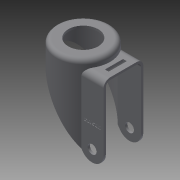
# Autodesk Inventor part: 2.05456.444-FORK
Saved by Autodesk Inventor 2014 SP2 (Build 180246200, 246)
## iProperties
Created: 2018-12-09
Part Number: 2.05456.444-FORK
Material: Generic
Catalog Web Link: www.cadenas.de
Description: 2 Series Stainless Steel Fork-Capacitiy up to 325 lbs Each
Vendor: COLSONGROUP
Document SubType Name: Modeling
Designer: psadmin
Manufacturer: COLSONGROUP
Mass: 30.1099 g
Surface Area: 255.342 cm^2
Volume: 30.1099 cm^3
Density: 1 g/cm^3
Appearance: PSOLRGB-175-175-175
Category: PARTsolutions
Company: COLSONGROUP
Title: 2.05456.444-FORK
Author: Cadenas PARTsolutions
Comments: Capacitiy up to 325 lbs Each
PSOL_IDENT_0: {$CADENAS_DATA\23d-libs\colsongroup\colson\casters\2_series_stainless_steel\2_series_stainless_steel
PSOL_IDENT_1: _fork.prj},210 {VTYP=3D},{NB=2.05456.444-FORK},{LINA=2.05456.444-FORK},{NN=2 Series Stainless Steel
PSOL_IDENT_2: Fork},{DATE=13.07.2017 07:15:58},{GEOMDATE=28.02.2017 12:04:00},{VERSION=},{LINEID=10},{WBVAR=MO,D,W
PSOL_IDENT_3: ,TT,BR},{WBNUMERIC=D,W}  {NB=2.05456.444-FORK},{LINA=2.05456.444-FORK},{KT=DUMMY},{PN=2.05456.444},{
PSOL_IDENT_4: SER=2 Series Stainless Steel},{MO=TPS},{MOPN=456},{SIZE=3 3/4\" x 2 3/4\"},{D=5.00000000},{DALG=3,3.
PSOL_IDENT_5: 5,4,5},{DPN=05},{W=1.25},{WALG=1.25,1.3125},{TT=PRFG},{TTALG= 'THT','ThermoTech', 'PLF','Polyolefin'
PSOL_IDENT_6: ,'PHI','Polyurethane HI-TECH','TPE','TPE High-Temp','PRFG','Performa Rubber (Flat)','TH','Thermo' },
PSOL_IDENT_7: {WTPN1=4},{WTPN3=},{WB=Derlin},{WBPN=44},{CAP=325},{BR=},{BRALG= '','None',' BRK1','Top Lock Brake (
PSOL_IDENT_8: BRK1)',' BRK2','Tech Lock Brake (BRK2)',' BRK4','Total Lock Brake (BRK4)' },{H=6.18750000},{R=4.0625
PSOL_IDENT_9: 0000},{WEIGHT=2.75000000},{FONTSIZE=0.12375},{MODEL=Swivel},{HEIGHT=2.75000},{WIDTH=3.75000},{HDY1=2
PSOL_IDENT_10: .81250},{HDY2=3.06250},{HDX1=1.75000},{HR=0.17000},{RR=0.5},{CP=0.53600},{X=1.25},{Y=-2.1515}
NN: 2 Series Stainless Steel Fork
NT: Capacitiy up to 325 lbs Each
NB: 2.05456.444-FORK
NBSYN: $PN.-FORK
LINA: 2.05456.444-FORK
SER: 2 Series Stainless Steel
MO: Top Plate Swivel
D: 5
W: 1.25
TT: Performa Rubber (Flat)
HDY1: 2.8125
HDY2: 3.0625
HDX1: 1.75
HR: 0.17
SUPPLIER: COLSONGROUP
ARTICLENO: 2.05456.444-FORK
BOMINFO: 2.05456.444-FORK
CREATOR: CADENAS GmbH
Autodesk Inventor part; units mm, degrees
sketch "Sketch_9" plane through (0, 0, 0) normal (1, 0, 0) x (0, 1, 0)
  line L0 (-15.494, 21.971) -> (-139.3508, 21.971)
  line L1 (-139.3508, 21.971) -> (-139.3508, -21.971)
  line L2 (-139.3508, -21.971) -> (-15.494, -21.971)
  arc A0 (-15.494, -21.971) -> (-8.382, -14.859) centre (-15.494, -14.859) ccw
  line L3 (-8.382, -14.859) -> (-8.382, 14.859)
  arc A1 (-8.382, 14.859) -> (-15.494, 21.971) centre (-15.494, 14.859) ccw
  constraints: 8 end point, 4 point on circle, 2 centre point
extrude "Extrusion1" add sketch "Sketch_9" along normal blind 45.72
sketch "Sketch_10" plane through (0, 0, 0) normal (0, 0, 1) x (1, 0, 0)
  line L0 (0, 0) -> (0, -130.9688)
  line L1 (0, -130.9688) -> (-29.591, -130.9688)
  line L2 (-29.591, -130.9688) -> (-29.591, -4.826)
  arc A0 (-24.765, 0) -> (-29.591, -4.826) centre (-24.765, -4.826) ccw
  line L3 (-24.765, 0) -> (0, 0)
  line L4 (0, 0) -> (0, -130.9688)
  constraints: 10 end point, 2 point on circle, 1 centre point
revolve "Revolution1" add sketch "Sketch_10" angle 360 about axis through (0, 0, 0) along (0, 1, 0)
sketch "Sketch_11" plane through (0, 0, 0) normal (0, 0, 1) x (1, 0, 0)
  line L0 (0, 0) -> (0, -130.9688)
  line L1 (0, -130.9688) -> (-27.051, -130.9688)
  line L2 (-27.051, -130.9688) -> (-27.051, -4.826)
  arc A0 (-24.765, -2.54) -> (-27.051, -4.826) centre (-24.765, -4.826) ccw
  line L3 (-24.765, -2.54) -> (-16.51, -2.54)
  line L4 (-16.51, -2.54) -> (-16.51, 0)
  line L5 (-16.51, 0) -> (0, 0)
  line L6 (0, 0) -> (0, -130.9688)
  constraints: 14 end point, 2 point on circle, 1 centre point
revolve "Revolution2" cut sketch "Sketch_11" angle 360 about axis through (0, 0, 0) along (0, 1, 0)
sketch "Sketch_12" plane through (0, 0, 0) normal (1, 0, 0) x (0, 1, 0)
  line L0 (-15.494, 19.431) -> (-141.8907, 19.431)
  line L1 (-141.8907, 19.431) -> (-141.8907, -19.431)
  line L2 (-141.8907, -19.431) -> (-15.494, -19.431)
  arc A0 (-15.494, -19.431) -> (-10.922, -14.859) centre (-15.494, -14.859) ccw
  line L3 (-10.922, -14.859) -> (-10.922, 14.859)
  arc A1 (-10.922, 14.859) -> (-15.494, 19.431) centre (-15.494, 14.859) ccw
  constraints: 8 end point, 4 point on circle, 2 centre point
extrude "Extrusion2" cut sketch "Sketch_12" along normal blind 50.8
sketch "Sketch_13" plane through (0, 0, 0) normal (0, 0, 1) x (1, 0, 0)
  line L0 (-42.291, -171.3865) -> (84.709, -171.3865)
  line L1 (84.709, -171.3865) -> (84.709, 0)
  line L2 (84.709, 0) -> (44.45, 0)
  line L3 (44.45, 0) -> (44.45, -80.0481)
  arc A0 (21.3298, -87.3083) -> (44.45, -80.0481) centre (31.75, -80.0481) ccw
  line L4 (21.3298, -87.3083) -> (-29.591, -14.224)
  line L5 (-29.591, -14.224) -> (-42.291, -14.224)
  line L6 (-42.291, -14.224) -> (-42.291, -171.3865)
  constraints: 14 end point, 2 point on circle, 1 centre point
extrude "Extrusion3" cut sketch "Sketch_13" along normal mid plane 101.6
sketch "Sketch_14" plane through (0, 0, 0) normal (0, 0, 1) x (1, 0, 0)
  circle A0 centre (31.75, -80.0481) radius 4.953
  constraints: 1 centre point
extrude "Extrusion4" cut sketch "Sketch_14" along normal mid plane 76.2
sketch "Sketch_15" plane through (0, -8.382, 0) normal (0, 1, 0) x (1, 0, 0)
  line L0 (34.036, 10.033) -> (34.036, -10.033)
  line L1 (34.036, -10.033) -> (38.1, -10.033)
  line L2 (38.1, -10.033) -> (38.1, 10.033)
  line L3 (38.1, 10.033) -> (34.036, 10.033)
  constraints: 8 end point
extrude "Extrusion5" cut sketch "Sketch_15" along normal mid plane 10.16
sketch "Sketch_31" plane through (0, 0, 21.971) normal (0, 0, 1) x (1, 0, 0)
  line L0 (21.59, -58.4581) -> (42.418, -58.4581)
  line L1 (42.418, -58.4581) -> (42.418, -50.8381)
  line L2 (42.418, -50.8381) -> (21.59, -50.8381)
  line L3 (21.59, -50.8381) -> (21.59, -58.4581)
  arc A0 (35.9216, -55.8222) -> (36.1042, -56.083) centre (36.1042, -55.8887) ccw
  line L4 (36.1042, -56.083) -> (36.2735, -56.083)
  arc A1 (36.2735, -56.083) -> (36.4561, -55.9551) centre (36.2735, -55.8887) ccw
  line L5 (36.4561, -55.9551) -> (37.0219, -54.4006)
  arc A2 (37.0219, -54.4006) -> (36.8393, -54.1398) centre (36.8393, -54.3341) ccw
  line L6 (36.8393, -54.1398) -> (36.67, -54.1398)
  arc A3 (36.67, -54.1398) -> (36.4874, -54.2677) centre (36.67, -54.3341) ccw
  line L7 (36.4874, -54.2677) -> (35.9216, -55.8222)
  arc A4 (27.3382, -55.8222) -> (27.5208, -56.083) centre (27.5208, -55.8887) ccw
  line L8 (27.5208, -56.083) -> (27.6902, -56.083)
  arc A5 (27.6902, -56.083) -> (27.8728, -55.9551) centre (27.6902, -55.8887) ccw
  line L9 (27.8728, -55.9551) -> (28.4386, -54.4006)
  arc A6 (28.4386, -54.4006) -> (28.256, -54.1398) centre (28.256, -54.3341) ccw
  line L10 (28.256, -54.1398) -> (28.0866, -54.1398)
  arc A7 (28.0866, -54.1398) -> (27.904, -54.2677) centre (28.0866, -54.3341) ccw
  line L11 (27.904, -54.2677) -> (27.3382, -55.8222)
  constraints: 24 end point, 16 point on circle, 8 centre point
extrude "Extrusion6" cut sketch "Sketch_31" along normal mid plane 1.016
sketch "Sketch_32" plane through (0, 0, 21.971) normal (0, 0, 1) x (1, 0, 0)
  line L0 (21.59, -58.4581) -> (42.418, -58.4581)
  line L1 (42.418, -58.4581) -> (42.418, -50.8381)
  line L2 (42.418, -50.8381) -> (21.59, -50.8381)
  line L3 (21.59, -50.8381) -> (21.59, -58.4581)
  line L4 (37.8579, -56.7307) -> (39.0239, -56.7307)
  line L5 (39.0239, -56.7307) -> (39.9204, -54.2677)
  arc A0 (40.103, -54.1398) -> (39.9204, -54.2677) centre (40.103, -54.3341) ccw
  line L6 (40.103, -54.1398) -> (40.2723, -54.1398)
  arc A1 (40.4549, -54.4006) -> (40.2723, -54.1398) centre (40.2723, -54.3341) ccw
  line L7 (40.4549, -54.4006) -> (39.6068, -56.7307)
  line L8 (39.6068, -56.7307) -> (40.7727, -56.7307)
  line L9 (40.7727, -56.7307) -> (41.7459, -54.0571)
  arc A2 (41.7459, -54.0571) -> (41.3502, -53.4921) centre (41.3502, -53.9131) ccw
  line L10 (41.3502, -53.4921) -> (40.4975, -53.4921)
  arc A3 (40.4975, -53.4921) -> (40.1018, -53.7691) centre (40.4975, -53.9131) ccw
  line L11 (40.1018, -53.7691) -> (40.2026, -53.4921)
  line L12 (40.2026, -53.4921) -> (39.0367, -53.4921)
  line L13 (39.0367, -53.4921) -> (37.8579, -56.7307)
  arc A4 (34.6306, -56.1657) -> (35.0263, -56.7307) centre (35.0263, -56.3097) ccw
  line L14 (35.0263, -56.7307) -> (37.045, -56.7307)
  arc A5 (37.045, -56.7307) -> (37.4406, -56.4537) centre (37.045, -56.3097) ccw
  line L15 (37.4406, -56.4537) -> (38.3129, -54.0571)
  arc A6 (38.3129, -54.0571) -> (37.9173, -53.4921) centre (37.9173, -53.9131) ccw
  line L16 (37.9173, -53.4921) -> (35.8985, -53.4921)
  arc A7 (35.8985, -53.4921) -> (35.5029, -53.7691) centre (35.8985, -53.9131) ccw
  line L17 (35.5029, -53.7691) -> (34.6306, -56.1657)
  arc A8 (31.1976, -56.1657) -> (31.5933, -56.7307) centre (31.5933, -56.3097) ccw
  line L18 (31.5933, -56.7307) -> (33.612, -56.7307)
  arc A9 (33.612, -56.7307) -> (34.0076, -56.4537) centre (33.612, -56.3097) ccw
  line L19 (34.0076, -56.4537) -> (34.3559, -55.4968)
  arc A10 (34.3559, -55.4968) -> (34.0189, -54.9358) centre (33.9603, -55.3528) ccw
  line L20 (34.0189, -54.9358) -> (33.1076, -54.8078)
  arc A11 (32.952, -54.5489) -> (33.1076, -54.8078) centre (33.1346, -54.6153) ccw
  line L21 (32.952, -54.5489) -> (33.0544, -54.2677)
  arc A12 (33.237, -54.1398) -> (33.0544, -54.2677) centre (33.237, -54.3341) ccw
  line L22 (33.237, -54.1398) -> (33.4064, -54.1398)
  arc A13 (33.589, -54.4006) -> (33.4064, -54.1398) centre (33.4064, -54.3341) ccw
  line L23 (33.589, -54.4006) -> (33.5189, -54.5932)
  line L24 (33.5189, -54.5932) -> (34.6848, -54.5932)
  line L25 (34.6848, -54.5932) -> (34.8799, -54.0571)
  arc A14 (34.8799, -54.0571) -> (34.4843, -53.4921) centre (34.4843, -53.9131) ccw
  line L26 (34.4843, -53.4921) -> (32.4656, -53.4921)
  arc A15 (32.4656, -53.4921) -> (32.0699, -53.7691) centre (32.4656, -53.9131) ccw
  line L27 (32.0699, -53.7691) -> (31.75, -54.6481)
  arc A16 (31.75, -54.6481) -> (32.087, -55.209) centre (32.1456, -54.7921) ccw
  line L28 (32.087, -55.209) -> (32.9983, -55.3371)
  arc A17 (33.1539, -55.596) -> (32.9983, -55.3371) centre (32.9713, -55.5295) ccw
  line L29 (33.1539, -55.596) -> (33.0232, -55.9551)
  arc A18 (32.8406, -56.083) -> (33.0232, -55.9551) centre (32.8406, -55.8887) ccw
  line L30 (32.8406, -56.083) -> (32.6712, -56.083)
  arc A19 (32.4886, -55.8222) -> (32.6712, -56.083) centre (32.6712, -55.8887) ccw
  line L31 (32.4886, -55.8222) -> (32.5587, -55.6296)
  line L32 (32.5587, -55.6296) -> (31.3928, -55.6296)
  line L33 (31.3928, -55.6296) -> (31.1976, -56.1657)
  line L34 (29.3079, -56.7307) -> (30.4738, -56.7307)
  line L35 (30.4738, -56.7307) -> (32.0062, -52.5205)
  line L36 (32.0062, -52.5205) -> (30.8403, -52.5205)
  line L37 (30.8403, -52.5205) -> (29.3079, -56.7307)
  arc A20 (26.0473, -56.1657) -> (26.4429, -56.7307) centre (26.4429, -56.3097) ccw
  line L38 (26.4429, -56.7307) -> (28.4616, -56.7307)
  arc A21 (28.4616, -56.7307) -> (28.8573, -56.4537) centre (28.4616, -56.3097) ccw
  line L39 (28.8573, -56.4537) -> (29.7296, -54.0571)
  arc A22 (29.7296, -54.0571) -> (29.3339, -53.4921) centre (29.3339, -53.9131) ccw
  line L40 (29.3339, -53.4921) -> (27.3152, -53.4921)
  arc A23 (27.3152, -53.4921) -> (26.9196, -53.7691) centre (27.3152, -53.9131) ccw
  line L41 (26.9196, -53.7691) -> (26.0473, -56.1657)
  arc A24 (22.6143, -56.1657) -> (23.0099, -56.7307) centre (23.0099, -56.3097) ccw
  line L42 (23.0099, -56.7307) -> (25.0286, -56.7307)
  arc A25 (25.0286, -56.7307) -> (25.4243, -56.4537) centre (25.0286, -56.3097) ccw
  line L43 (25.4243, -56.4537) -> (25.795, -55.4353)
  line L44 (25.795, -55.4353) -> (24.629, -55.4353)
  line L45 (24.629, -55.4353) -> (24.4398, -55.9551)
  arc A26 (24.2572, -56.083) -> (24.4398, -55.9551) centre (24.2572, -55.8887) ccw
  line L46 (24.2572, -56.083) -> (24.0878, -56.083)
  arc A27 (23.9052, -55.8222) -> (24.0878, -56.083) centre (24.0878, -55.8887) ccw
  line L47 (23.9052, -55.8222) -> (24.4711, -54.2677)
  arc A28 (24.6537, -54.1398) -> (24.4711, -54.2677) centre (24.6537, -54.3341) ccw
  line L48 (24.6537, -54.1398) -> (24.823, -54.1398)
  arc A29 (25.0056, -54.4006) -> (24.823, -54.1398) centre (24.823, -54.3341) ccw
  line L49 (25.0056, -54.4006) -> (24.8648, -54.7875)
  line L50 (24.8648, -54.7875) -> (26.0307, -54.7875)
  line L51 (26.0307, -54.7875) -> (26.2966, -54.0571)
  arc A30 (26.2966, -54.0571) -> (25.9009, -53.4921) centre (25.9009, -53.9131) ccw
  line L52 (25.9009, -53.4921) -> (23.8822, -53.4921)
  arc A31 (23.8822, -53.4921) -> (23.4866, -53.7691) centre (23.8822, -53.9131) ccw
  line L53 (23.4866, -53.7691) -> (22.6143, -56.1657)
  constraints: 108 end point, 64 point on circle, 32 centre point
extrude "Extrusion7" add sketch "Sketch_32" along normal mid plane 1.016
sketch "Sketch_30" plane through (31.75, 0, 0) normal (1, 0, 0) x (0, 0, -1)
  line L0 (-47.371, -146.4627) -> (-21.971, -146.4627)
  line L1 (-21.971, -146.4627) -> (-21.971, -15.494)
  line L2 (-21.971, -15.494) -> (-47.371, -15.494)
  line L3 (-47.371, -15.494) -> (-47.371, -146.4627)
  constraints: 8 end point
extrude "Extrusion8" cut sketch "Sketch_30" along normal mid plane 22.86
ref_plane "to_axle_XY" through (31.75, -80.0481, 21.971) normal (0, 0, 1) x (1, 0, 0)
ref_plane "to_axle_YZ" through (31.75, -80.0481, 21.971) normal (1, 0, 0) x (0, 1, 0)
ref_plane "to_axle_ZX" through (31.75, -80.0481, 21.971) normal (0, 1, 0) x (0, 0, 1)
ref_plane "to_brk2_XY" through (31.75, -80.0481, 0) normal (0, 0, 1) x (1, 0, 0)
ref_plane "to_brk2_YZ" through (31.75, -80.0481, 0) normal (1, 0, 0) x (0, 1, 0)
ref_plane "to_brk2_ZX" through (31.75, -80.0481, 0) normal (0, 1, 0) x (0, 0, 1)
ref_plane "to_brk4_XY" through (28.7528, -21.3868, 0) normal (0, 0, 1) x (1, 0, 0)
ref_plane "to_brk4_YZ" through (28.7528, -21.3868, 0) normal (1, 0, 0) x (0, 1, 0)
ref_plane "to_brk4_ZX" through (28.7528, -21.3868, 0) normal (0, 1, 0) x (0, 0, 1)
ref_plane "to_dummy_XY" through (0, 13.6144, 0) normal (0, -1, 0) x (1, 0, 0)
ref_plane "to_dummy_YZ" through (0, 13.6144, 0) normal (1, 0, 0) x (0, 0, 1)
ref_plane "to_dummy_ZX" through (0, 13.6144, 0) normal (0, 0, 1) x (0, -1, 0)
ref_plane "to_nut_XY" through (31.75, -80.0481, -21.971) normal (0, 0, 1) x (1, 0, 0)
ref_plane "to_nut_YZ" through (31.75, -80.0481, -21.971) normal (1, 0, 0) x (0, 1, 0)
ref_plane "to_nut_ZX" through (31.75, -80.0481, -21.971) normal (0, 1, 0) x (0, 0, 1)
ref_plane "to_wheel_XY" through (31.75, -80.0481, 0) normal (0, 0, -1) x (1, 0, 0)
ref_plane "to_wheel_YZ" through (31.75, -80.0481, 0) normal (1, 0, 0) x (0, -1, 0)
ref_plane "to_wheel_ZX" through (31.75, -80.0481, 0) normal (0, -1, 0) x (0, 0, -1)
body "Solid1"
